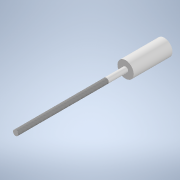
# Autodesk Inventor part: lead screw 160
Saved by Autodesk Inventor 2020 (Build 240168000, 168)
## iProperties
Created: 2020-07-02
Part Number: lead screw 160
Material: Generic
Document SubType Name: Modeling
Designer: Ashiqrahman
Density: 1 g/cm^3
Appearance: Default
Author: Ashiqrahman
Autodesk Inventor part; units mm, degrees
ref_plane "YZ Plane" through (0, 0, 0) normal (1, 0, 0) x (0, 1, 0)
ref_plane "XZ Plane" through (0, 0, 0) normal (0, 1, 0) x (-1, 0, 0)
ref_plane "XY Plane" through (0, 0, 0) normal (0, 0, 1) x (1, 0, 0)
sketch "Sketch1" plane through (0, 0, 0) normal (0, 0, 1) x (1, 0, 0)
  circle A0 centre (0, 0) radius 4
  dimension "d0" = 8
  constraints: 1 centre point, 1 coincident
  measures "d0" diameter of A0
extrude "Extrusion1" add sketch "Sketch1" along normal blind 170
thread "Thread1" size "M8x1.25" class "6g" standard "ANSI Metric M Profile" length 140
body "Solid1"
